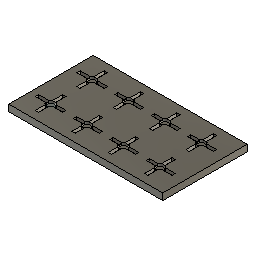
fold lines v5 (Autodesk Fusion 360 design; units mm, degrees)
Autodesk Fusion 360 part; units mm, degrees
note: some values were not read from the file. Chosen so that the rebuilt part matches the saved one: which face or edge a step refers to; a direction; which pieces of a blend or face edit are solid. Set by a fixed rule: which sketch regions a step uses.
sketch "Sketch1" plane through (0, 0, 0) normal (0, 0, 1) x (1, 0, 0)
  line L0 (0, 0) -> (200, 0)
  line L1 (200, 0) -> (200, 80)
  line L2 (200, 80) -> (0, 80)
  line L3 (0, 80) -> (0, 0)
  dimension "d1" = 200
  dimension "d2" = 80
  constraint horizontal L0
  constraint vertical L1
  constraint horizontal L2
  constraint vertical L3
  constraint coincident L0.start L3.end
  measures "d1" distance of L0.start L0.end
  measures "d2" distance of L0.start L2.end
extrude "Extrude1" add sketch "Sketch1" along normal blind 4 makes body 1
sketch "Sketch3" plane through (0, 0, 4) normal (0, 0, 1) x (-1, 0, 0)
  line L0 (0, -80) -> (0, 0)
  line L1 (0, 0) -> (-200, 0)
  line L2 (-200, 0) -> (-200, -80)
  line L3 (-200, -80) -> (0, -80)
  circle A0 centre (-17.3, -14) radius 2.5
  dimension "d9" = 5
  measures "d9" diameter of A0
extrude "Extrude3" cut sketch "Sketch3" against normal blind 1.5 draft -15 contours A0 bodies 1
sketch "Sketch4" plane through (0, 0, 4) normal (0, 0, 1) x (-1, 0, 0)
  line L0 (0, -80) -> (0, 0)
  line L1 (0, 0) -> (-200, 0)
  line L2 (-200, 0) -> (-200, -80)
  line L3 (-200, -80) -> (0, -80)
  line L4 (-20, -15) -> (-26, -15)
  line L5 (-26, -15) -> (-26, -13)
  line L6 (-26, -13) -> (-20, -13)
  line L7 (-20, -13) -> (-20, -15)
  circle A0 centre (-17.3, -14) radius 2.5
  dimension "d12" = 6
  dimension "d13" = 2
  constraint horizontal L4
  constraint vertical L5
  constraint horizontal L6
  constraint vertical L7
  measures "d12" distance of L4.start L4.end
  measures "d13" distance of L4.start L6.end
extrude "Extrude4" cut sketch "Sketch4" against normal blind 1.5 draft -15 contours L4 L5 L6 L7 bodies 1
move_face "MoveFace1" by (-0.38, 0, 0) 2 faces at (20.134, 13.8006, 3.5) (25.866, 14.1994, 3.5) on bodies 1
sketch "Sketch5" plane through (0, 0, 4) normal (0, 0, 1) x (-1, 0, 0)
  arc A0 (-19.62, -14.9315) -> (-19.62, -13.0685) centre (-17.3, -14) ccw
  line L0 (-19.62, -14.9315) -> (-19.62, -15)
  line L1 (-19.62, -15) -> (-25.62, -15)
  line L2 (-25.62, -15) -> (-25.62, -13)
  line L3 (-25.62, -13) -> (-19.62, -13)
  line L4 (-19.62, -13) -> (-19.62, -13.0685)
  line L5 (0, -80) -> (0, 0)
  line L6 (0, 0) -> (-200, 0)
  line L7 (-200, 0) -> (-200, -80)
  line L8 (-200, -80) -> (0, -80)
  line L9 (-3.915, -15.0266) -> (-13.915, -15.0266)
  line L10 (-13.915, -15.0266) -> (-13.915, -13.0266)
  line L11 (-13.915, -13.0266) -> (-3.915, -13.0266)
  line L12 (-3.915, -13.0266) -> (-3.915, -15.0266)
  dimension "d16" = 10
  dimension "d17" = 2
  constraint horizontal L9
  constraint vertical L10
  constraint horizontal L11
  constraint vertical L12
  measures "d16" distance of L9.start L9.end
  measures "d17" distance of L9.start L11.end
extrude "Extrude5" cut sketch "Sketch5" against normal blind 1.5 draft -15 contours L9 L10 L11 L12 bodies 1
delete_face "DeleteFace1" 5 faces at (10.4477, 14.226, 2.5) (7.3823, 14.8927, 3.5) (4.049, 14.226, 3.5) (10.4477, 13.1606, 3.5) (13.781, 14.226, 3.5) on bodies 1
move_face "MoveFace3" by (-0.05, 0, 0) 2 faces at (19.9178, 13.9748, 2.8888) (25.486, 14.1994, 3.5) on bodies 1
pattern_circular "C-Pattern2" count 4 over 360 about axis through (17.3, 14, 4) along (0, 0, -1) of 5 faces at (21.704, 14.1994, 2.5) (23.4431, 14.866, 3.5) (19.8762, 13.985, 2.8572) (23.4431, 13.134, 3.5) (25.436, 14.1994, 3.5) on bodies 1
sketch "Sketch14" plane through (0, 9.9442, -2.6646) normal (0, -0.965926, 0.258819) x (1, 0, 0)
  line L0 (17.8981, 5.3467) -> (18.2871, 6.85)
  spline S0 degree 2 poles (18.2871, 6.85) (17.3, 6.0607) (16.3129, 6.85) knots 0.006548 0.006548 0.006548 0.221006 0.221006 0.221006
  line L1 (16.3129, 6.85) -> (16.7019, 5.3467)
  line L2 (16.7019, 5.3467) -> (17.8981, 5.3467)
  line L3 (16.3129, 6.85) -> (16.1124, 7.6245)
  line L4 (18.4876, 7.6245) -> (18.2871, 6.85)
  line L5 (16.3129, 6.85) -> (18.2871, 6.85)
  line L6 (18.4876, 7.6245) -> (16.1124, 7.6245)
  line L7 (18.4876, 7.6245) -> (18.2871, 6.85)
  dimension "d50" = 0.8
  constraint coincident S0.end L1.start
  constraint coincident L1 L3.end
  constraint coincident L0 L4.start
  constraint coincident L0.end S0.start
  constraint parallel L0 L4
  constraint parallel L5 L6
  measures "d50" distance of S0.end L3.end
extrude "Extrude9" cut sketch "Sketch14" against normal blind 0.6 contours L3 L4 L5 L6 L7 bodies 1
sketch "Sketch15" plane through (0, 0, 2.5) normal (0, 0, 1) x (-1, 0, 0)
  circle A0 centre (-17.3, -14) radius 2.0981
sketch "Sketch16" plane through (19.2591, 0, 5.1604) normal (0.965926, 0, 0.258819) x (0, 1, 0)
  line L0 (14.5981, -2.7543) -> (14.9871, -1.2511)
  spline S0 degree 2 poles (14.9871, -1.2511) (14, -2.0404) (13.0129, -1.2511) knots 0.415953 0.415953 0.415953 0.753319 0.753319 0.753319
  line L1 (13.0129, -1.2511) -> (13.4019, -2.7543)
  line L2 (13.4019, -2.7543) -> (14.5981, -2.7543)
  line L3 (13.0129, -1.2511) -> (13.2133, -2.0255)
  line L4 (13.2133, -2.0255) -> (14.7867, -2.0255)
  line L5 (14.7867, -2.0255) -> (14.9871, -1.2511)
  line L6 (14.9871, -1.2511) -> (13.0129, -1.2511)
  dimension "d53" = 0.8
  constraint coincident S0.end L1.start
  constraint coincident L1 L3.end
  constraint coincident L0 L4.end
  constraint horizontal L4
  constraint coincident L0.end S0.start
  measures "d53" distance of S0.end L3.end
extrude "Extrude10" cut sketch "Sketch16" against normal blind 0.5 contours L0 S0 L1 L3 L4 L5 bodies 1
sketch "Sketch17" plane through (13.0232, 0, -3.4896) normal (-0.965926, 0, 0.258819) x (0, -1, 0)
  line L0 (-13.4019, 6.2008) -> (-13.0129, 7.7041)
  spline S0 degree 2 poles (-13.0129, 7.7041) (-14, 6.9148) (-14.9871, 7.7041) knots 0.006548 0.006548 0.006548 0.221006 0.221006 0.221006
  line L1 (-14.9871, 7.7041) -> (-14.5981, 6.2008)
  line L2 (-14.5981, 6.2008) -> (-13.4019, 6.2008)
  line L3 (-14.9871, 7.7041) -> (-14.7867, 6.9296)
  line L4 (-14.7867, 6.9296) -> (-13.2133, 6.9296)
  line L5 (-13.2133, 6.9296) -> (-13.0129, 7.7041)
  line L6 (-13.0129, 7.7041) -> (-14.9871, 7.7041)
  dimension "d56" = 0.8
  constraint coincident S0.end L1.start
  constraint parallel L1 L3
  constraint coincident L0 L4.end
  constraint horizontal L4
  constraint coincident L0.end S0.start
  measures "d56" distance of S0.end L3.end
extrude "Extrude11" cut sketch "Sketch17" against normal blind 0.7 contours L0 S0 L1 L3 L4 L5 bodies 1
fillet "Fillet5" radius 0.05 5 edges at (19.5715, 14, 3.1472) (15.0669, 14.4006, 3.1369) (15.0669, 13.5994, 3.1369) (14.8167, 14, 3.2039) (19.7833, 14, 3.2039) on bodies 1
move_face "OffsetFaces5" offset -9 1 faces at (0, 53.3333, 1.3333) on bodies 1
move_face "OffsetFaces6" offset -1 1 faces at (72.6667, 0, 1.3333) on bodies 1
move_face "OffsetFaces7" offset -168 1 faces at (200, 27.3333, 1.3333) on bodies 1
move_face "OffsetFaces8" offset -53 1 faces at (24.3333, 80, 2.6667) on bodies 1
copy_body "CopyPasteBodies4" bodies 1 makes body 2
move_body "Move4" bodies 2 to x (1, 0, 0) y (0, 1, 0) z (0, 0, 1) at (22, 0, 0)
copy_body "CopyPasteBodies5" bodies 1 2 makes body 3 makes body 4
move_body "Move5" bodies 3 4 to x (1, 0, 0) y (0, 1, 0) z (0, 0, 1) at (44, 0, 0)
copy_body "CopyPasteBodies6" bodies 4 2 1 3 makes body 5 makes body 6 makes body 7 makes body 8
move_body "Move6" bodies 5 6 7 8 to x (1, 0, 0) y (0, 1, 0) z (0, 0, 1) at (0, 25, 0)
combine "Combine2" operation add target body 1 tool bodies 3 8 2 7 6 4 5
move_face "OffsetFaces9" offset 4 1 faces at (9, 35, 1.3333) on bodies 1
